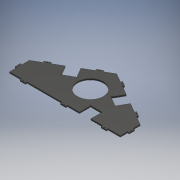
# Autodesk Inventor part: BA19
Saved by Autodesk Inventor 2017 (Build 210142000, 142)
## iProperties
Created: 2019-06-03
Part Number: BA19
Material: Polyethylene, High Density
Document SubType Name: Modeling
Designer: Dell
Density: 0.952 g/cm^3
Appearance: Smooth - Black
Mass: 405.553 g
Surface Area: 1476.06 cm^2
Volume: 426.001 cm^3
Author: Dell
Autodesk Inventor part; units mm, degrees
ref_plane "YZ Plane" through (0, 0, 0) normal (1, 0, 0) x (0, 1, 0)
ref_plane "XZ Plane" through (0, 0, 0) normal (0, 1, 0) x (-1, 0, 0)
ref_plane "XY Plane" through (0, 0, 0) normal (0, 0, 1) x (1, 0, 0)
sketch "Sketch1" plane through (0, 0, 0) normal (0, 0, 1) x (1, 0, 0)
  line L0 (0, 303.5592) -> (262.89, 151.7796) construction
  line L1 (262.89, 151.7796) -> (262.89, -151.7796) construction
  line L2 (262.89, -151.7796) -> (0, -303.5592) construction
  line L3 (0, -303.5592) -> (-262.89, -151.7796) construction
  line L4 (-262.89, -151.7796) -> (-262.89, 151.7796) construction
  line L5 (-262.89, 151.7796) -> (0, 303.5592) construction
  line L6 (0, 296.2269) -> (256.54, 148.1134)
  line L7 (256.54, 148.1134) -> (256.54, -148.1134)
  line L8 (256.54, -148.1134) -> (0, -296.2269)
  line L9 (0, -296.2269) -> (-256.54, -148.1134)
  line L10 (-256.54, -148.1134) -> (-256.54, 148.1134)
  line L11 (-256.54, 148.1134) -> (0, 296.2269)
  line L12 (-256.54, 56.5296) -> (256.54, 56.5296)
  line L13 (256.54, 148.1134) -> (256.54, 56.5296)
  line L14 (-256.54, 56.5296) -> (-256.54, 148.1134)
  point P0 (0, 0)
  point P1 (0, 0)
  point P2 (-256.54, 0)
  dimension "d0" = 525.78
  dimension "d1" = 6.35
  dimension "d2" = 95.25
  constraints: 30 end point, 2 collinear, 2 point on line, 1 coincident, 1 horizontal alignment, 1 midpoint, 1 perpendicular, 18 other
  measures "d0" distance between parallel lines of L1 L4
  measures "d1" distance between parallel lines of L5 L11
  measures "d2" distance from line of L4.end L12
extrude "Extrusion1" add sketch "Sketch1" along normal blind 6.35 contours L6 L7 L12 L10 L11
sketch "Sketch2" plane through (0, 0, 6.35) normal (0, 0, 1) x (1, 0, 0)
  line L0 (-256.54, 56.5296) -> (256.54, 56.5296) projected
  line L1 (-200.2, 56.5296) -> (-174.8, 56.5296)
  line L2 (-174.8, 56.5296) -> (-174.8, 48.9096)
  line L3 (-174.8, 48.9096) -> (-200.2, 48.9096)
  line L4 (-200.2, 48.9096) -> (-200.2, 56.5296)
  line L5 (12.7, 56.5296) -> (-12.7, 56.5296)
  line L6 (-12.7, 56.5296) -> (-12.7, 48.9096)
  line L7 (-12.7, 48.9096) -> (12.7, 48.9096)
  line L8 (12.7, 48.9096) -> (12.7, 56.5296)
  line L9 (174.8, 56.5296) -> (200.2, 56.5296)
  line L10 (200.2, 56.5296) -> (200.2, 48.9096)
  line L11 (200.2, 48.9096) -> (174.8, 48.9096)
  line L12 (174.8, 48.9096) -> (174.8, 56.5296)
  line L13 (-256.54, 148.1134) -> (-256.54, 56.5296) projected
  line L14 (-187.5, 48.9096) -> (187.5, 48.9096) construction
  point P0 (0, 0)
  point P1 (0, 56.5296)
  point P2 (0, 48.9096)
  point P3 (0, 56.5296)
  dimension "d5" = 25.4
  dimension "d7" = 25.4
  dimension "d8" = 25.4
  dimension "d13" = 7.62
  dimension "d47" = 375
  constraints: 26 end point, 6 midpoint, 6 parallel, 4 point on line, 3 horizontal, 3 perpendicular, 1 horizontal alignment, 1 vertical alignment
  measures "d5" distance of L2.end L3.end
  measures "d7" distance of L6.end L7.end
  measures "d8" distance of L10.end L11.end
  measures "d13" distance of L3.end L1.start
  measures "d47" distance of L14.start L14.end
extrude "Extrusion2" add sketch "Sketch2" against normal blind 6.35
sketch "Sketch3" plane through (0, 0, 6.35) normal (0, 0, 1) x (1, 0, 0)
  line L0 (256.54, 56.5296) -> (256.54, 148.1134) projected
  line L1 (256.54, 115.0215) -> (264.16, 115.0215)
  line L2 (264.16, 115.0215) -> (264.16, 89.6215)
  line L3 (264.16, 89.6215) -> (256.54, 89.6215)
  line L4 (256.54, 89.6215) -> (256.54, 115.0215)
  line L5 (-256.54, 148.1134) -> (-256.54, 56.5296) projected
  line L6 (-256.54, 89.6215) -> (-264.16, 89.6215)
  line L7 (-264.16, 89.6215) -> (-264.16, 115.0215)
  line L8 (-264.16, 115.0215) -> (-256.54, 115.0215)
  line L9 (-256.54, 115.0215) -> (-256.54, 89.6215)
  point P0 (0, 0)
  point P1 (256.54, 102.3215)
  point P2 (-256.54, 102.3215)
  dimension "d16" = 25.4
  dimension "d17" = 25.4
  dimension "d18" = 7.62
  dimension "d19" = 7.62
  constraints: 16 end point, 4 midpoint, 4 parallel, 2 horizontal, 2 perpendicular, 2 point on line
  measures "d16" distance of L6.end L7.end
  measures "d17" distance of L1.end L2.end
  measures "d18" distance of L6.start L6.end
  measures "d19" distance of L2.end L3.end
extrude "Extrusion3" add sketch "Sketch3" against normal blind 6.35
sketch "Sketch4" plane through (0, 0, 6.35) normal (0, 0, 1) x (1, 0, 0)
  line L0 (256.54, 148.1134) -> (0, 296.2269) projected
  line L1 (40.2818, 272.9702) -> (62.2789, 260.2702)
  line L2 (62.2789, 260.2702) -> (66.0889, 266.8693)
  line L3 (66.0889, 266.8693) -> (44.0918, 279.5693)
  line L4 (44.0918, 279.5693) -> (40.2818, 272.9702)
  line L5 (194.2611, 184.0702) -> (216.2582, 171.3702)
  line L6 (216.2582, 171.3702) -> (220.0682, 177.9693)
  line L7 (220.0682, 177.9693) -> (198.0711, 190.6693)
  line L8 (198.0711, 190.6693) -> (194.2611, 184.0702)
  line L9 (256.54, 148.1134) -> (0, 296.2269) projected
  line L10 (0, 296.2269) -> (0, 363.4216)
  line L11 (-256.54, 148.1134) -> (0, 296.2269)
  line L12 (-40.2818, 272.9702) -> (-62.2789, 260.2702)
  line L13 (-62.2789, 260.2702) -> (-66.0889, 266.8693)
  line L14 (-66.0889, 266.8693) -> (-44.0918, 279.5693)
  line L15 (-44.0918, 279.5693) -> (-40.2818, 272.9702)
  line L16 (-194.2611, 184.0702) -> (-216.2582, 171.3702)
  line L17 (-216.2582, 171.3702) -> (-220.0682, 177.9693)
  line L18 (-220.0682, 177.9693) -> (-198.0711, 190.6693)
  line L19 (-198.0711, 190.6693) -> (-194.2611, 184.0702)
  line L20 (-256.54, 148.1134) -> (0, 296.2269)
  line L21 (66.0889, 266.8693) -> (198.0711, 190.6693)
  line L22 (132.08, 228.7693) -> (128.27, 222.1702)
  point P0 (0, 0)
  dimension "d22" = 25.4
  dimension "d23" = 25.4
  dimension "d26" = 7.62
  dimension "d27" = 7.62
  dimension "d30" = 152.4
  constraints: 42 end point, 9 symmetric about line, 8 point on line, 4 parallel, 3 perpendicular, 2 midpoint, 1 vertical
  measures "d22" distance of L2.end L3.end
  measures "d23" distance of L6.end L7.end
  measures "d26" distance of L5.end L6.end
  measures "d27" distance of L1.end L2.end
  measures "d30" distance of L2.end L7.end
extrude "Extrusion4" add sketch "Sketch4" against normal blind 6.35 contours L0 L8 L7 L6 | L0 L4 L3 L2 | L17 L18 L19 L11 | L13 L14 L15 L11
sketch "Sketch6" plane through (0, 0, 6.35) normal (0, 0, 1) x (1, 0, 0)
  line L0 (12.7, 56.5296) -> (174.8, 56.5296) projected
  line L1 (68.35, 56.5296) -> (119.15, 56.5296)
  line L2 (119.15, 56.5296) -> (119.15, 107.3296)
  line L3 (119.15, 107.3296) -> (68.35, 107.3296)
  line L4 (68.35, 107.3296) -> (68.35, 56.5296)
  line L5 (256.54, 56.5296) -> (256.54, 89.6215) projected
  line L6 (194.2611, 184.0702) -> (62.2789, 260.2702) projected
  line L7 (105.1731, 235.5052) -> (79.1381, 190.4112)
  line L8 (79.1381, 190.4112) -> (125.3319, 163.7412)
  line L9 (125.3319, 163.7412) -> (151.3669, 208.8352)
  line L10 (151.3669, 208.8352) -> (105.1731, 235.5052)
  line L11 (-62.2789, 260.2702) -> (-194.2611, 184.0702) projected
  line L12 (-105.1731, 235.5052) -> (-79.1381, 190.4112)
  line L13 (-79.1381, 190.4112) -> (-125.3319, 163.7412)
  line L14 (-125.3319, 163.7412) -> (-151.3669, 208.8352)
  line L15 (-151.3669, 208.8352) -> (-105.1731, 235.5052)
  line L16 (67.08, 56.5296) -> (120.42, 56.5296)
  line L17 (120.42, 56.5296) -> (120.42, 108.5996)
  line L18 (120.42, 108.5996) -> (67.08, 108.5996)
  line L19 (67.08, 108.5996) -> (67.08, 56.5296)
  line L20 (12.7, 56.5296) -> (174.8, 56.5296) projected
  point P0 (0, 0)
  point P1 (-59.69, 56.5296)
  point P2 (8.89, 56.5296)
  point P3 (128.27, 222.1702)
  point P4 (-128.27, 222.1702)
  point P5 (34.29, 56.5296)
  dimension "d31" = 188.19
  dimension "d32" = 50.8
  dimension "d33" = 50.8
  dimension "d34" = 53.34
  dimension "d35" = 52.07
  dimension "d36" = 52.07
  dimension "d37" = 53.34
  dimension "d38" = 1.27
  dimension "d39" = 1.27
  dimension "d40" = 1.27
  constraints: 32 end point, 8 parallel, 6 perpendicular, 4 midpoint, 4 point on line, 2 horizontal
  measures "d31" distance between parallel lines of L5 L4
  measures "d32" distance of L2.end L3.end
  measures "d33" distance of L1.end L2.end
  measures "d34" distance of L7.end L8.end
  measures "d35" distance of L7.start L7.end
  measures "d36" distance of L12.start L12.end
  measures "d37" distance of L12.end L13.end
  measures "d38" distance between parallel lines of L4 L19
  measures "d39" distance between parallel lines of L2 L17
  measures "d40" distance between parallel lines of L3 L18
extrude "Extrusion5" cut sketch "Sketch6" against normal through all
sketch "Sketch7" plane through (0, 0, 6.35) normal (0, 0, 1) x (1, 0, 0)
  circle A0 centre (0, 174.2957) radius 60
  point P0 (0, 0)
  point P1 (0, 296.2269)
  dimension "d43" = 120
  dimension "d44" = 121.9312
  constraints: 1 centre point, 1 vertical alignment
  measures "d43" diameter of A0
  measures "d44" distance of A0.centre point (0, 296.227)
extrude "Extrusion6" cut sketch "Sketch7" against normal through all
sketch "Sketch8" plane through (0, 0, 6.35) normal (0, 0, 1) x (1, 0, 0)
  circle A0 centre (-187.5, 52.7196) radius 2.25
  circle A1 centre (-260.35, 102.3215) radius 2.25
  circle A2 centre (-207.1647, 181.0197) radius 2.25
  circle A3 centre (0, 52.7196) radius 2.25
  circle A4 centre (187.5, 52.7196) radius 2.25
  circle A5 centre (-53.1853, 269.9197) radius 2.25
  circle A6 centre (260.35, 102.3215) radius 2.25
  line L0 (-200.2, 48.9096) -> (-174.8, 48.9096) projected
  line L1 (-256.54, 115.0215) -> (-264.16, 115.0215) projected
  line L2 (-12.7, 48.9096) -> (12.7, 48.9096) projected
  line L3 (174.8, 48.9096) -> (200.2, 48.9096) projected
  line L4 (264.16, 115.0215) -> (256.54, 115.0215) projected
  line L5 (-264.16, 115.0215) -> (-264.16, 89.6215) projected
  line L6 (264.16, 89.6215) -> (264.16, 115.0215) projected
  line L7 (200.2, 48.9096) -> (200.2, 56.5296) projected
  line L8 (12.7, 48.9096) -> (12.7, 56.5296) projected
  line L9 (-174.8, 48.9096) -> (-174.8, 56.5296) projected
  line L10 (-216.2582, 171.3702) -> (-220.0682, 177.9693) projected
  line L11 (-218.1632, 174.6697) -> (-207.1647, 181.0197) construction
  line L12 (-207.1647, 181.0197) -> (-209.0697, 184.3193) construction
  line L13 (-198.0711, 190.6693) -> (-220.0682, 177.9693) projected
  line L14 (-66.0889, 266.8693) -> (-62.2789, 260.2702) projected
  line L15 (-64.1839, 263.5697) -> (-53.1853, 269.9197) construction
  line L16 (-53.1853, 269.9197) -> (-55.0903, 273.2193) construction
  line L17 (-44.0918, 279.5693) -> (-66.0889, 266.8693) projected
  line L18 (40.2818, 272.9702) -> (0, 296.2269) projected
  line L19 (0, 296.2269) -> (0, 343.5756)
  circle A7 centre (207.1647, 181.0197) radius 2.25
  circle A8 centre (53.1853, 269.9197) radius 2.25
  line L20 (216.2582, 171.3702) -> (220.0682, 177.9693)
  line L21 (218.1632, 174.6697) -> (207.1647, 181.0197) construction
  line L22 (207.1647, 181.0197) -> (209.0697, 184.3193) construction
  line L23 (198.0711, 190.6693) -> (220.0682, 177.9693)
  line L24 (66.0889, 266.8693) -> (62.2789, 260.2702)
  line L25 (64.1839, 263.5697) -> (53.1853, 269.9197) construction
  line L26 (53.1853, 269.9197) -> (55.0903, 273.2193) construction
  line L27 (44.0918, 279.5693) -> (66.0889, 266.8693)
  point P0 (0, 0)
  point P1 (-187.5, 48.9096)
  point P2 (-260.35, 115.0215)
  point P3 (0, 48.9096)
  point P4 (187.5, 48.9096)
  point P5 (260.35, 115.0215)
  point P6 (-264.16, 102.3215)
  point P7 (264.16, 102.3215)
  point P8 (200.2, 52.7196)
  point P9 (12.7, 52.7196)
  point P10 (-174.8, 52.7196)
  dimension "d48" = 4.5
  dimension "d49" = 4.5
  dimension "d50" = 4.5
  dimension "d51" = 4.5
  dimension "d52" = 4.5
  dimension "d53" = 4.5
  dimension "d56" = 4.5
  constraints: 26 end point, 14 midpoint, 12 symmetric about line, 9 centre point, 5 horizontal alignment, 5 vertical alignment, 4 perpendicular, 1 vertical, 2 other
  measures "d48" diameter of A0
  measures "d49" diameter of A1
  measures "d50" diameter of A2
  measures "d51" diameter of A3
  measures "d52" diameter of A4
  measures "d53" diameter of A5
  measures "d56" diameter of A6
extrude "Extrusion7" cut sketch "Sketch8" against normal through all
sketch "Sketch9" plane through (0, 0, 6.35) normal (0, 0, 1) x (1, 0, 0)
  circle A0 centre (207.1647, 181.0197) radius 2.25 construction
  circle A1 centre (-53.1853, 269.9197) radius 2.25 construction
  circle A2 centre (0, 52.7196) radius 2.25 construction
  circle A3 centre (-260.35, 102.3215) radius 2.25 construction
  circle A4 centre (-187.5, 52.7196) radius 2.25 construction
  circle A5 centre (-207.1647, 181.0197) radius 2.25 construction
  circle A6 centre (187.5, 52.7196) radius 2.25 construction
  circle A7 centre (260.35, 102.3215) radius 2.25 construction
  circle A8 centre (53.1853, 269.9197) radius 2.25 construction
  circle A9 centre (0, 174.2957) radius 60 construction
  line L0 (-125.3319, 163.7412) -> (-151.3669, 208.8352) construction
  line L1 (-151.3669, 208.8352) -> (-194.2611, 184.0702) construction
  line L2 (-194.2611, 184.0702) -> (-198.0711, 190.6693) construction
  line L3 (-198.0711, 190.6693) -> (-220.0682, 177.9693) construction
  line L4 (-220.0682, 177.9693) -> (-216.2582, 171.3702) construction
  line L5 (-216.2582, 171.3702) -> (-256.54, 148.1134) construction
  line L6 (-256.54, 148.1134) -> (-256.54, 115.0215) construction
  line L7 (-256.54, 115.0215) -> (-264.16, 115.0215) construction
  line L8 (-264.16, 115.0215) -> (-264.16, 89.6215) construction
  line L9 (-264.16, 89.6215) -> (-256.54, 89.6215) construction
  line L10 (-256.54, 89.6215) -> (-256.54, 56.5296) construction
  line L11 (-256.54, 56.5296) -> (-200.2, 56.5296) construction
  line L12 (-200.2, 56.5296) -> (-200.2, 48.9096) construction
  line L13 (-200.2, 48.9096) -> (-174.8, 48.9096) construction
  line L14 (-174.8, 48.9096) -> (-174.8, 56.5296) construction
  line L15 (-174.8, 56.5296) -> (-12.7, 56.5296) construction
  line L16 (-12.7, 56.5296) -> (-12.7, 48.9096) construction
  line L17 (-12.7, 48.9096) -> (12.7, 48.9096) construction
  line L18 (12.7, 48.9096) -> (12.7, 56.5296) construction
  line L19 (12.7, 56.5296) -> (67.08, 56.5296) construction
  line L20 (67.08, 56.5296) -> (67.08, 108.5996) construction
  line L21 (67.08, 108.5996) -> (120.42, 108.5996) construction
  line L22 (120.42, 108.5996) -> (120.42, 56.5296) construction
  line L23 (120.42, 56.5296) -> (174.8, 56.5296) construction
  line L24 (174.8, 56.5296) -> (174.8, 48.9096) construction
  line L25 (174.8, 48.9096) -> (200.2, 48.9096) construction
  line L26 (200.2, 48.9096) -> (200.2, 56.5296) construction
  line L27 (200.2, 56.5296) -> (256.54, 56.5296) construction
  line L28 (256.54, 56.5296) -> (256.54, 89.6215) construction
  line L29 (256.54, 89.6215) -> (264.16, 89.6215) construction
  line L30 (264.16, 89.6215) -> (264.16, 115.0215) construction
  line L31 (264.16, 115.0215) -> (256.54, 115.0215) construction
  line L32 (256.54, 115.0215) -> (256.54, 148.1134) construction
  line L33 (256.54, 148.1134) -> (216.2582, 171.3702) construction
  line L34 (216.2582, 171.3702) -> (220.0682, 177.9693) construction
  line L35 (220.0682, 177.9693) -> (198.0711, 190.6693) construction
  line L36 (198.0711, 190.6693) -> (194.2611, 184.0702) construction
  line L37 (194.2611, 184.0702) -> (151.3669, 208.8352) construction
  line L38 (151.3669, 208.8352) -> (125.3319, 163.7412) construction
  line L39 (125.3319, 163.7412) -> (79.1381, 190.4112) construction
  line L40 (79.1381, 190.4112) -> (105.1731, 235.5052) construction
  line L41 (105.1731, 235.5052) -> (62.2789, 260.2702) construction
  line L42 (62.2789, 260.2702) -> (66.0889, 266.8693) construction
  line L43 (66.0889, 266.8693) -> (44.0918, 279.5693) construction
  line L44 (44.0918, 279.5693) -> (40.2818, 272.9702) construction
  line L45 (40.2818, 272.9702) -> (0, 296.2269) construction
  line L46 (0, 296.2269) -> (-40.2818, 272.9702) construction
  line L47 (-40.2818, 272.9702) -> (-44.0918, 279.5693) construction
  line L48 (-44.0918, 279.5693) -> (-66.0889, 266.8693) construction
  line L49 (-66.0889, 266.8693) -> (-62.2789, 260.2702) construction
  line L50 (-62.2789, 260.2702) -> (-105.1731, 235.5052) construction
  line L51 (-105.1731, 235.5052) -> (-79.1381, 190.4112) construction
  line L52 (-79.1381, 190.4112) -> (-125.3319, 163.7412) construction
  line L53 (-108.2399, 236.3269) -> (-65.3457, 261.0919) construction
  line L54 (-65.3457, 261.0919) -> (-69.1557, 267.691) construction
  line L55 (-69.1557, 267.691) -> (-43.2701, 282.6361) construction
  line L56 (-43.2701, 282.6361) -> (-39.4601, 276.037) construction
  line L57 (-39.4601, 276.037) -> (0, 298.8193) construction
  line L58 (0, 298.8193) -> (39.4601, 276.037) construction
  line L59 (39.4601, 276.037) -> (43.2701, 282.6361) construction
  line L60 (43.2701, 282.6361) -> (69.1557, 267.691) construction
  line L61 (69.1557, 267.691) -> (65.3457, 261.0919) construction
  line L62 (65.3457, 261.0919) -> (108.2399, 236.3269) construction
  line L63 (108.2399, 236.3269) -> (82.2049, 191.233) construction
  line L64 (82.2049, 191.233) -> (124.5101, 166.808) construction
  line L65 (124.5101, 166.808) -> (150.5451, 211.902) construction
  line L66 (150.5451, 211.902) -> (193.4394, 187.137) construction
  line L67 (193.4394, 187.137) -> (197.2494, 193.7361) construction
  line L68 (197.2494, 193.7361) -> (223.135, 178.791) construction
  line L69 (223.135, 178.791) -> (219.325, 172.1919) construction
  line L70 (219.325, 172.1919) -> (258.7851, 149.4096) construction
  line L71 (258.7851, 149.4096) -> (258.7851, 117.2666) construction
  line L72 (258.7851, 117.2666) -> (266.4051, 117.2666) construction
  line L73 (266.4051, 117.2666) -> (266.4051, 87.3765) construction
  line L74 (266.4051, 87.3765) -> (258.7851, 87.3765) construction
  line L75 (258.7851, 87.3765) -> (258.7851, 54.2845) construction
  line L76 (258.7851, 54.2845) -> (202.4451, 54.2845) construction
  line L77 (202.4451, 54.2845) -> (202.4451, 46.6645) construction
  line L78 (202.4451, 46.6645) -> (172.5549, 46.6645) construction
  line L79 (172.5549, 46.6645) -> (172.5549, 54.2845) construction
  line L80 (172.5549, 54.2845) -> (118.1749, 54.2845) construction
  line L81 (118.1749, 54.2845) -> (118.1749, 106.3545) construction
  line L82 (118.1749, 106.3545) -> (69.3251, 106.3545) construction
  line L83 (69.3251, 106.3545) -> (69.3251, 54.2845) construction
  line L84 (69.3251, 54.2845) -> (14.9451, 54.2845) construction
  line L85 (14.9451, 54.2845) -> (14.9451, 46.6645) construction
  line L86 (14.9451, 46.6645) -> (-14.9451, 46.6645) construction
  line L87 (-14.9451, 46.6645) -> (-14.9451, 54.2845) construction
  line L88 (-14.9451, 54.2845) -> (-172.5549, 54.2845) construction
  line L89 (-172.5549, 54.2845) -> (-172.5549, 46.6645) construction
  line L90 (-172.5549, 46.6645) -> (-202.4451, 46.6645) construction
  line L91 (-202.4451, 46.6645) -> (-202.4451, 54.2845) construction
  line L92 (-202.4451, 54.2845) -> (-258.7851, 54.2845) construction
  line L93 (-258.7851, 54.2845) -> (-258.7851, 87.3765) construction
  line L94 (-258.7851, 87.3765) -> (-266.4051, 87.3765) construction
  line L95 (-266.4051, 87.3765) -> (-266.4051, 117.2666) construction
  line L96 (-266.4051, 117.2666) -> (-258.7851, 117.2666) construction
  line L97 (-258.7851, 117.2666) -> (-258.7851, 149.4096) construction
  line L98 (-258.7851, 149.4096) -> (-219.325, 172.1919) construction
  line L99 (-219.325, 172.1919) -> (-223.135, 178.791) construction
  line L100 (-223.135, 178.791) -> (-197.2494, 193.7361) construction
  line L101 (-197.2494, 193.7361) -> (-193.4394, 187.137) construction
  line L102 (-193.4394, 187.137) -> (-150.5451, 211.902) construction
  line L103 (-150.5451, 211.902) -> (-124.5101, 166.808) construction
  line L104 (-124.5101, 166.808) -> (-82.2049, 191.233) construction
  line L105 (-82.2049, 191.233) -> (-108.2399, 236.3269) construction
  circle A10 centre (-258.7851, 87.3765) radius 3.175
  circle A11 centre (-258.7851, 117.2666) radius 3.175
  line L106 (-220.0682, 177.9693) -> (-216.2582, 171.3702) projected
  circle A12 centre (-219.325, 172.1919) radius 3.175
  circle A13 centre (-193.4394, 187.137) radius 3.175
  circle A14 centre (-124.5101, 166.808) radius 3.175
  circle A15 centre (-82.2049, 191.233) radius 3.175
  circle A16 centre (-65.3457, 261.0919) radius 3.175
  circle A17 centre (-39.4601, 276.037) radius 3.175
  line L107 (40.2818, 272.9702) -> (0, 296.2269) projected
  circle A18 centre (39.4601, 276.037) radius 3.175
  circle A19 centre (65.3457, 261.0919) radius 3.175
  line L108 (79.1381, 190.4112) -> (125.3319, 163.7412) projected
  circle A20 centre (82.2049, 191.233) radius 3.175
  circle A21 centre (124.5101, 166.808) radius 3.175
  line L109 (194.2611, 184.0702) -> (151.3669, 208.8352) projected
  circle A22 centre (193.4394, 187.137) radius 3.175
  line L110 (256.54, 148.1134) -> (216.2582, 171.3702) projected
  circle A23 centre (219.325, 172.1919) radius 3.175
  line L111 (256.54, 115.0215) -> (256.54, 148.1134) projected
  circle A24 centre (258.7851, 117.2666) radius 3.175
  circle A25 centre (258.7851, 87.3765) radius 3.175
  circle A26 centre (202.4451, 54.2845) radius 3.175
  line L112 (120.42, 56.5296) -> (174.8, 56.5296) projected
  circle A27 centre (172.5549, 54.2845) radius 3.175
  circle A28 centre (118.1749, 106.3545) radius 3.175
  circle A29 centre (69.3251, 106.3545) radius 3.175
  circle A30 centre (14.9451, 54.2845) radius 3.175
  circle A31 centre (-14.9451, 54.2845) radius 3.175
  line L113 (-174.8, 56.5296) -> (-12.7, 56.5296) projected
  circle A32 centre (-172.5549, 54.2845) radius 3.175
  line L114 (-256.54, 56.5296) -> (-200.2, 56.5296) projected
  circle A33 centre (-202.4451, 54.2845) radius 3.175
  point P0 (0, 0)
  dimension "d59" = 6.35
  constraints: 106 end point, 23 coincident, 124 other
extrude "Extrusion8" cut sketch "Sketch9" against normal through all
equation "\"d1\" = Panel_Thickness"
equation "\"d3\" = Panel_Thickness"
equation "\"d13\" = Panel_Thickness + Fit_Tolerance"
equation "\"d14\" = Panel_Thickness"
equation "\"d18\" = Panel_Thickness + Fit_Tolerance"
equation "\"d19\" = Panel_Thickness + Fit_Tolerance"
equation "\"d20\" = Panel_Thickness"
equation "\"d26\" = Panel_Thickness + Fit_Tolerance"
equation "\"d27\" = Panel_Thickness + Fit_Tolerance"
equation "\"d28\" = Panel_Thickness"
equation "\"d38\" = Fit_Tolerance"
equation "\"d39\" = d38"
equation "\"d40\" = Fit_Tolerance"
equation "\"d59\" = Tool_Dia"
equation "\"Panel_Thickness\" = 6.35"
equation "\"Fit_Tolerance\" = 1.27"
equation "\"Tool_Dia\" = 6.35"
body "Solid1"
